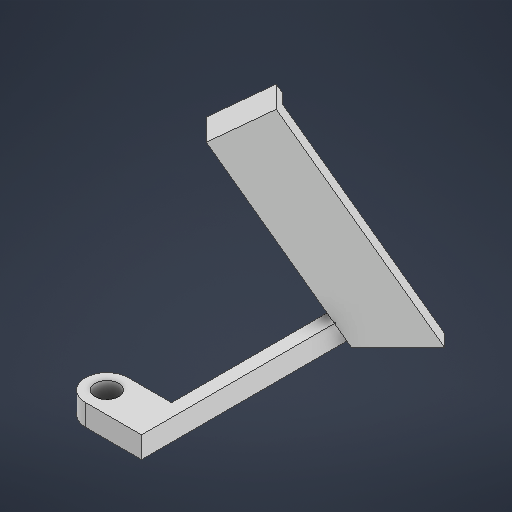
# Autodesk Inventor part: Pixy2 mount
Saved by Autodesk Inventor 2026 (Build 300175050, 175E)
## iProperties
Created: 2025-10-30
Part Number: Pixy2 mount
Material: Generic
Document SubType Name: Modeling
Designer: aduwa
Density: 1 g/cm^3
Appearance: Default
Author: aduwa
Autodesk Inventor part; units mm, degrees
ref_plane "YZ Plane" through (0, 0, 0) normal (1, 0, 0) x (0, 1, 0)
ref_plane "XZ Plane" through (0, 0, 0) normal (0, 1, 0) x (-1, 0, 0)
ref_plane "XY Plane" through (0, 0, 0) normal (0, 0, 1) x (1, 0, 0)
sketch "Sketch2" plane through (0, 0, 0) normal (0, 1, 0) x (-1, 0, 0)
  circle A0 centre (13.1, 80.1) radius 2.75
  circle A1 centre (80.1, 13.1) radius 2.75 construction
  line L0 (13.1, 80.1) -> (13.1, 13.1)
  line L1 (13.1, 13.1) -> (80.1, 13.1)
  line L2 (3, 37.224) -> (37.224, 3)
  line L3 (3, 37.224) -> (51.4, 37.224) construction
  circle A2 centre (80.1, 13.1) radius 2.75
  line L4 (3.1, 112.1) -> (3.1, 79.1)
  line L5 (79.1, 3.1) -> (112.1, 3.1)
  circle A3 centre (13.1, 80.1) radius 5
  line L6 (13.1, 75.1) -> (3, 75.1)
  line L7 (3, 75.1) -> (3, 3)
  line L8 (13.1, 85.1) -> (0, 85.1)
  line L9 (0, 85.1) -> (0, 0)
  circle A4 centre (80.1, 13.1) radius 5
  line L10 (85.1, 13.1) -> (85.1, 0)
  line L11 (75.1, 13.1) -> (75.1, 3)
  line L12 (75.1, 3) -> (3, 3)
  line L13 (85.1, 0) -> (0, 0)
  line L14 (3, 37.224) -> (-4.0711, 30.1529)
  line L15 (3, 37.224) -> (13, 37.224) construction
  point P0 (0, 0)
  point P1 (0, 34.224)
  dimension "d11" = 48.4
  dimension "d12" = 45
  dimension "d13" = 10
  dimension "d14" = 10.1
  dimension "d15" = 13.1
  dimension "d16" = 3
  dimension "d17" = 10
  dimension "d18" = 13.1
  dimension "d19" = 10.1
  dimension "d20" = 10
  dimension "d21" = 135
  constraints: 32 end point, 8 perpendicular, 5 centre point, 4 point on circle, 4 point on line, 4 tangent, 2 coincident, 2 equal length, 2 horizontal, 1 parallel, 1 vertical
  measures "d11" distance of L2.start L2.end
  measures "d12" angle of L2 L3
  measures "d13" diameter of A3
  measures "d14" distance of L6.start L6.end
  measures "d15" distance of L8.start L8.end
  measures "d16" distance between parallel lines of L9 L7
  measures "d17" diameter of A4
  measures "d18" distance of L10.start L10.end
  measures "d19" distance of L11.start L11.end
  measures "d20" distance of L2.start L14.end
  measures "d21" angle of L14 L15
extrude "Extrusion2" add sketch "Sketch2" along normal blind 5 contours L6 L7 L14 L9 L8 A3 | A3
sketch "Sketch4" plane through (-3, 0, 37.224) normal (-0.7071068, 0, -0.7071068) x (-0.7071068, 0, 0.7071068)
  line L0 (0, 0) -> (0, 5) projected
  line L1 (0, 5) -> (20.05, 39.7276)
  line L2 (0, 5) -> (40.1, 5) construction
  line L3 (8.5319, 46.3776) -> (-11.5181, 11.65)
  line L4 (-11.5181, 11.65) -> (0, 5)
  line L5 (8.5319, 46.3776) -> (20.05, 39.7276)
  line L6 (-4.2426, 0) -> (0, 0) projected
  line L7 (0, 0) -> (0, 5) projected
  line L8 (-4.2426, 5) -> (0, 5) projected
  line L9 (-4.2426, 0) -> (-4.2426, 5) projected
  line L10 (-4.2426, 5) -> (-4.2426, 7.4495)
  point P0 (-28.4426, 0)
  dimension "d33" = 300
  dimension "d34" = 40.1
  dimension "d35" = 13.3
  constraints: 12 end point, 2 perpendicular, 1 equal length, 1 horizontal, 1 point on line, 1 vertical
  measures "d34" distance of L0.end L1.end
  measures "d35" distance of L1.end L3.start
extrude "Extrusion3" add sketch "Sketch4" against normal blind 4 contours L4 L3 L5 L1
sketch "Sketch6" plane through (0, -2.3485, 34.224) normal (-0.7071068, 0, -0.7071068) x (-0.7071068, 0, 0.7071068)
  line L0 (0, 2.3485) -> (0, 7.3485) projected
  circle A0 centre (0.9836, 15.0036) radius 2.6
  line L1 (3.7898, 7.6099) -> (-7.6418, 14.2099)
  circle A1 centre (6.9836, 25.3959) radius 2.6
  line L2 (0, 2.3485) -> (4.2426, 2.3485) projected
  line L3 (-7.2755, 13.9985) -> (4.2426, 7.3485) projected
  line L4 (11.0336, 32.4107) -> (-8.7344, -1.8285)
  line L5 (4.2426, 2.3485) -> (4.2426, 7.3485) projected
  line L6 (0, 7.3485) -> (4.2426, 7.3485) projected
  point P0 (-24.2, 2.3485)
  dimension "d38" = 5.2
  dimension "d39" = 5
  dimension "d40" = 12
  constraints: 4 end point, 2 centre point, 2 point on line, 1 collinear, 1 equal radius
  measures "d38" diameter of A0
  measures "d39" distance from line of L1 A0.centre
  measures "d40" distance of A1.centre A0.centre
extrude "Extrusion5" [suppressed]
fillet "Fillet1" [suppressed]
sketch "Sketch9" plane through (-0.1716, 0, 40.0524) normal (0.7071068, 0, 0.7071068) x (0.7071068, 0, -0.7071068)
  line L0 (0, 5) -> (-20.05, 39.7276) projected
  line L1 (-20.05, 39.7276) -> (-12.55, 26.7372)
  line L2 (-12.55, 26.7372) -> (-15.1481, 25.2372)
  line L3 (-15.1481, 25.2372) -> (-22.6481, 38.2276)
  line L4 (-22.6481, 38.2276) -> (-20.05, 39.7276)
  line L5 (-8.5319, 46.3776) -> (-20.05, 39.7276) projected
  line L6 (-14.2909, 43.0526) -> (11.2, -1.0989)
  line L7 (-8.5319, 46.3776) -> (-1.0319, 33.3872)
  line L8 (1.5662, 34.8872) -> (-5.9338, 47.8776)
  line L9 (-1.0319, 33.3872) -> (1.5662, 34.8872)
  line L10 (-5.9338, 47.8776) -> (-8.5319, 46.3776)
  point P0 (28.4426, 0)
  point P1 (4.6202, -0.5061)
  point P2 (4.1955, 0)
  dimension "d46" = 15
  dimension "d47" = 3
  constraints: 18 end point, 4 perpendicular, 3 symmetric about line, 1 midpoint, 2 other
  measures "d46" distance of L1.start L1.end
  measures "d47" distance of L1.end L2.end
extrude "Extrusion6" [suppressed]
sketch "Sketch10" plane through (-17.1775, 39.7276, 51.4015) normal (-0.3535534, 0.8660254, 0.3535534) x (0.7071068, 0, 0.7071068)
  line L0 (0, 0) -> (0, 13.3) projected
  line L1 (0, 0) -> (4, 0) projected
  line L2 (4, 13.3) -> (4, 0) projected
  line L3 (0, 13.3) -> (4, 13.3) projected
  line L4 (-0.6, 8.15) -> (0, 8.15)
  line L5 (0, -1.85) -> (0, 5.15)
  line L6 (0, 5.15) -> (-0.6, 5.15)
  arc A0 (-0.6, 5.15) -> (-1.099, 4.6815) centre (-0.6, 4.65) ccw
  arc A1 (-1.7225, 4.2287) -> (-1.099, 4.6815) centre (-1.598, 4.713) ccw
  arc A2 (-1.7225, 9.0713) -> (-1.7225, 4.2287) centre (-1.1, 6.65) ccw
  arc A3 (-1.099, 8.6185) -> (-1.7225, 9.0713) centre (-1.598, 8.587) ccw
  arc A4 (-1.099, 8.6185) -> (-0.6, 8.15) centre (-0.6, 8.65) ccw
  line L7 (0, 0) -> (0, 13.3) projected
  line L8 (0.6, 5.35) -> (-0.6, 5.35)
  arc A5 (-0.6, 5.35) -> (-1.2986, 4.6941) centre (-0.6, 4.65) ccw
  arc A6 (-1.6727, 4.4224) -> (-1.2986, 4.6941) centre (-1.598, 4.713) ccw
  arc A7 (-1.6727, 8.8776) -> (-1.6727, 4.4224) centre (-1.1, 6.65) ccw
  arc A8 (-1.2986, 8.6059) -> (-1.6727, 8.8776) centre (-1.598, 8.587) ccw
  arc A9 (-1.2986, 8.6059) -> (-0.6, 7.95) centre (-0.6, 8.65) ccw
  line L9 (-0.6, 7.95) -> (0.6, 7.95)
  line L10 (0.3, -1.85) -> (0.3, 5.45)
  line L11 (0.3, 5.45) -> (-0.6, 5.45)
  arc A10 (-0.6, 5.45) -> (-1.3984, 4.7004) centre (-0.6, 4.65) ccw
  arc A11 (-1.6478, 4.5193) -> (-1.3984, 4.7004) centre (-1.598, 4.713) ccw
  arc A12 (-1.6478, 8.7807) -> (-1.6478, 4.5193) centre (-1.1, 6.65) ccw
  arc A13 (-1.3984, 8.5996) -> (-1.6478, 8.7807) centre (-1.598, 8.587) ccw
  arc A14 (-1.3984, 8.5996) -> (-0.6, 7.85) centre (-0.6, 8.65) ccw
  line L12 (-0.6, 7.85) -> (0.4, 7.85)
  line L13 (0.4, -1.85) -> (0.4, 5.55)
  line L14 (0.4, 5.55) -> (-0.6, 5.55)
  arc A15 (-0.6, 5.55) -> (-1.4982, 4.7067) centre (-0.6, 4.65) ccw
  arc A16 (-1.6229, 4.6161) -> (-1.4982, 4.7067) centre (-1.598, 4.713) ccw
  arc A17 (-1.6229, 8.6839) -> (-1.6229, 4.6161) centre (-1.1, 6.65) ccw
  arc A18 (-1.4982, 8.5933) -> (-1.6229, 8.6839) centre (-1.598, 8.587) ccw
  arc A19 (-1.4982, 8.5933) -> (-0.6, 7.75) centre (-0.6, 8.65) ccw
  line L15 (-0.6, 7.75) -> (0.4, 7.75)
  point P0 (-24.2, 22.132)
  point P1 (-11.4165, -11.1867)
  point P2 (0, 6.65)
  point P3 (0, 6.65)
  point P4 (0, 5.35)
  point P5 (0, 7.95)
  point P6 (0, 5.45)
  point P7 (0, 7.85)
  point P8 (0, 5.55)
  point P9 (0, 7.75)
  dimension "d64" = 2.5
  dimension "d65" = 0.6
  dimension "d66" = 1.1
  dimension "d67" = 0.2
  dimension "d68" = 0.3
  dimension "d69" = 0.4
  constraints: 40 point on circle, 22 end point, 20 centre point, 2 midpoint, 1 collinear, 1 horizontal alignment, 1 parallel, 20 other
  measures "d64" radius of A2
  measures "d65" distance of L5.end L6.end
  measures "d66" distance from line of L5 A2.centre
  measures "d67" radial gap between concentric circles of A2 A7
  measures "d68" radial gap between concentric circles of A2 A12
  measures "d69" radial gap between concentric circles of A2 A17
extrude "Extrusion7" add sketch "Sketch10" against normal up to surface (40.1 mm away) contours L14 A15 A16 A17 A18 A19 L15 L0
sketch "Sketch11" plane through (-14.3491, 39.7276, 54.2299) normal (-0.3535534, 0.8660254, 0.3535534) x (0.7071068, 0, 0.7071068)
  line L0 (-4, 7.75) -> (-4, 13.3) projected
  line L1 (-4, 0) -> (0, 0) projected
  line L2 (0, 13.3) -> (0, 0) projected
  line L3 (-4, 13.3) -> (0, 13.3) projected
  line L4 (0, 0) -> (0, 13.3)
  line L5 (0, 0) -> (-7.3, 0)
  line L6 (-7.7, 13.3) -> (0, 13.3)
  line L7 (0, 13.3) -> (0, 0)
  line L8 (-4, 0) -> (-4, 5.55) projected
  line L9 (-4, 7.75) -> (-4.6, 7.75) projected
  arc A0 (-5.4982, 8.5933) -> (-4.6, 7.75) centre (-4.6, 8.65) ccw projected
  arc A1 (-5.4982, 8.5933) -> (-5.6229, 8.6839) centre (-5.598, 8.587) ccw projected
  arc A2 (-5.6229, 8.6839) -> (-5.6229, 4.6161) centre (-5.1, 6.65) ccw projected
  arc A3 (-5.6229, 4.6161) -> (-5.4982, 4.7067) centre (-5.598, 4.713) ccw projected
  arc A4 (-4.6, 5.55) -> (-5.4982, 4.7067) centre (-4.6, 4.65) ccw projected
  line L10 (-4.6, 5.55) -> (-4, 5.55) projected
  line L11 (-7.2, 13.3) -> (-7.2, 0)
  arc A5 (-5.6229, 8.6839) -> (-5.6229, 4.6161) centre (-5.1, 6.65) ccw projected
  point P0 (-28.2, 22.132)
  point P1 (-4, 0)
  point P2 (0, 13.3)
  point P3 (0, 0)
  point P4 (-4, 13.3)
  point P5 (0, 0)
  point P6 (-4, 13.3)
  point P7 (-4, 0)
  point P8 (-7.2, 6.65)
  point P9 (-7.2, 6.65)
  point P10 (-4, 0)
  constraints: 10 end point, 1 horizontal, 1 midpoint, 1 parallel, 1 perpendicular, 1 point on circle, 1 point on line, 1 tangent
extrude "Extrusion8" add sketch "Sketch11" along normal blind 2
sketch "Sketch12" plane through (7.973, 11.65, 31.9078) normal (0.3535534, -0.8660254, -0.3535534) x (0.7071068, 0, 0.7071068)
  line L0 (31.9748, 40.7808) -> (-4, 9.6258) projected
  line L1 (-4, 0) -> (-4, 5.55) projected
  line L2 (-4, 0) -> (0, 0) projected
  line L3 (0, 13.3) -> (0, 0) projected
  line L4 (-4, 13.3) -> (0, 13.3) projected
  line L5 (-4, 7.75) -> (-4, 13.3) projected
  line L6 (-4.6, 7.75) -> (-4, 7.75) projected
  arc A0 (-5.4982, 8.5933) -> (-4.6, 7.75) centre (-4.6, 8.65) ccw projected
  arc A1 (-5.4982, 8.5933) -> (-5.6229, 8.6839) centre (-5.598, 8.587) ccw projected
  arc A2 (-5.6229, 8.6839) -> (-5.6229, 4.6161) centre (-5.1, 6.65) ccw projected
  arc A3 (-5.6229, 4.6161) -> (-5.4982, 4.7067) centre (-5.598, 4.713) ccw projected
  arc A4 (-4.6, 5.55) -> (-5.4982, 4.7067) centre (-4.6, 4.65) ccw projected
  line L7 (-4, 5.55) -> (-4.6, 5.55) projected
  point P0 (-28.2, -8.832)
extrude "Extrusion9" add sketch "Sketch12" along normal up to surface surface through (-9.05, 0, 59.662) normal (0, 1, 0)
body "Solid2"
